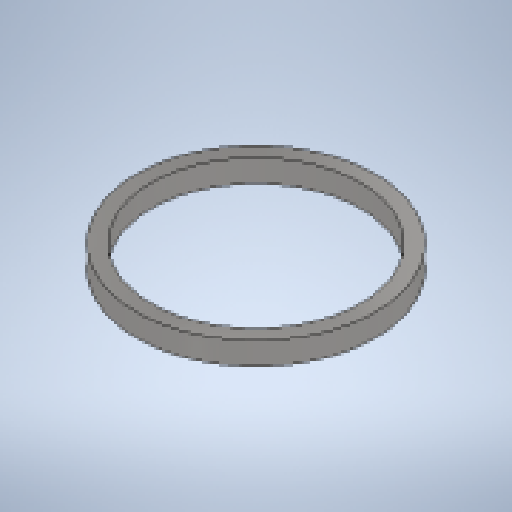
# Autodesk Inventor part: Ring
Saved by Autodesk Inventor 2023.4 (Build 274418000, 418)
## iProperties
Created: 2024-04-30
Part Number: Ring
Material: Stainless Steel
Document SubType Name: Modeling
Designer: Nathan Cai
Mass: 154.444 g
Surface Area: 101.341 cm^2
Volume: 19.3056 cm^3
Density: 8 g/cm^3
Appearance: Semi-Polished
Author: Nathan Cai
Autodesk Inventor part; units mm, degrees
ref_plane "YZ Plane" through (0, 0, 0) normal (1, 0, 0) x (0, 1, 0)
ref_plane "XZ Plane" through (0, 0, 0) normal (0, 1, 0) x (-1, 0, 0)
ref_plane "XY Plane" through (0, 0, 0) normal (0, 0, 1) x (1, 0, 0)
sketch "Sketch1" plane through (0, 0, 0) normal (0, 1, 0) x (-1, 0, 0)
  circle A0 centre (0, 0) radius 47.625
  circle A1 centre (0, 0) radius 53.975
  dimension "d0" = 95.25
  dimension "d4" = 6.35
  constraints: 2 centre point, 2 coincident
  measures "d0" diameter of A0
  measures "d4" radial gap between concentric circles of A0 A1
extrude "Extrusion1" add sketch "Sketch1" along normal blind 9.525
body "Solid1"
